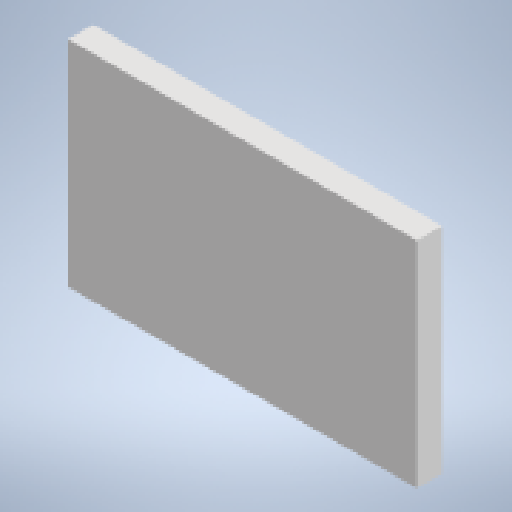
# Autodesk Inventor part: Mattress2
Saved by Autodesk Inventor 2024 (Build 280153000, 153)
## iProperties
Created: 2024-10-17
Part Number: Mattress2
Material: 一般
Document SubType Name: Modeling
Designer: jerry
Density: 1 g/cm^3
Appearance: 預設
Author: jerry
Autodesk Inventor part; units mm, degrees
ref_plane "YZ Plane" through (0, 0, 0) normal (1, 0, 0) x (0, 1, 0)
ref_plane "XZ Plane" through (0, 0, 0) normal (0, 1, 0) x (-1, 0, 0)
ref_plane "XY Plane" through (0, 0, 0) normal (0, 0, 1) x (1, 0, 0)
sketch "草圖1" plane through (0, 0, 0) normal (0, 0, 1) x (1, 0, 0)
  line L0 (1600, 400) -> (300, 400)
  line L1 (300, 400) -> (300, -400)
  line L2 (300, -400) -> (1600, -400)
  line L3 (1600, -400) -> (1600, 400)
  line L4 (1600, 400) -> (300, -400) construction
  line L5 (300, 400) -> (1600, -400) construction
  point P0 (0, 0)
  point P1 (950, 0)
  dimension "d1" = 1300
  dimension "d2" = 800
  constraints: 12 end point, 2 midpoint, 2 parallel, 1 horizontal, 1 perpendicular
  measures "d1" distance of L2.end L1.end
  measures "d2" distance of L1.end L0.end
extrude "擠出1" add sketch "草圖1" against normal blind 100
fillet "圓角1" radius 10 4 edges at (950, 400, -100) (300, 0, -100) (950, -400, -100) (1600, 0, -100)
